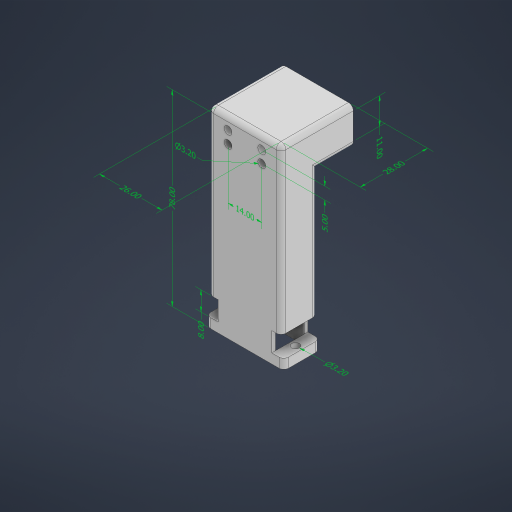
# Autodesk Inventor part: attachment of brush
Saved by Autodesk Inventor 2024.2 (Build 282272000, 272)
## iProperties
Created: 2024-03-09
Part Number: attachment of brush
Material: Generic
Document SubType Name: Modeling
Designer: seifs
Density: 1 g/cm^3
Appearance: Default
Author: seifs
Autodesk Inventor part; units mm, degrees
ref_plane "YZ Plane" through (0, 0, 0) normal (1, 0, 0) x (0, 1, 0)
ref_plane "XZ Plane" through (0, 0, 0) normal (0, 1, 0) x (-1, 0, 0)
ref_plane "XY Plane" through (0, 0, 0) normal (0, 0, 1) x (1, 0, 0)
sketch "Sketch1" plane through (0, 0, 0) normal (0, 0, 1) x (1, 0, 0)
  line L0 (-15, 7.5) -> (15, 7.5)
  line L1 (15, 7.5) -> (15, -7.5)
  line L2 (15, -7.5) -> (-15, -7.5)
  line L3 (-15, -7.5) -> (-15, 7.5)
  line L4 (-15, 7.5) -> (15, -7.5) construction
  line L5 (15, 7.5) -> (-15, -7.5) construction
  line L6 (-15, 0) -> (-7, 0) construction
  line L7 (-7, 0) -> (-7, -2.5) construction
  line L8 (0, 7.5) -> (0, -7.5) construction
  circle A0 centre (-7, -2.5) radius 1.6
  line L9 (0, -7.5) -> (0, 7.5) construction
  circle A1 centre (-7, 2.5) radius 1.6
  circle A2 centre (7, -2.5) radius 1.6
  circle A3 centre (7, 2.5) radius 1.6
  line L10 (7, 2.5) -> (-7, 2.5) construction
  point P0 (0, 0)
  dimension "d0" = 30
  dimension "d1" = 15
  dimension "d3" = 2.5
  dimension "d4" = 3.2
  dimension "d11" = 14
  constraints: 22 end point, 5 midpoint, 5 symmetric about line, 4 centre point, 3 horizontal, 2 parallel, 2 perpendicular, 1 coincident, 3 other
  measures "d0" distance of L1.end L2.end
  measures "d1" distance of L0.end L1.end
  measures "d3" distance of L6.end L7.end
  measures "d4" diameter of A0
  measures "d11" distance of L10.start L10.end
extrude "Extrusion1" add sketch "Sketch1" along normal blind 30
sketch "Sketch2" plane through (-15, -7.5, 0) normal (0, -1, 0) x (1, 0, 0)
  line L0 (0, 30) -> (30, 30) projected
  line L1 (0, 30) -> (30, 30)
  line L2 (30, 30) -> (30, 15)
  line L3 (30, 15) -> (0, 15)
  line L4 (0, 15) -> (0, 30)
  point P0 (15, 0)
  dimension "d7" = 30
  dimension "d8" = 15
  constraints: 8 end point, 2 parallel, 1 horizontal, 1 perpendicular
  measures "d7" distance of L2.end L3.end
  measures "d8" distance of L1.end L2.end
extrude "Extrusion2" add sketch "Sketch2" along normal blind 50
sketch "Sketch3" plane through (-15, -57.5, 0) normal (0, -1, 0) x (1, 0, 0)
  line L0 (0, 15) -> (30, 15) projected
  line L1 (15, 15) -> (15, 22.5) construction
  line L2 (15, 22.5) -> (3.85, 22.5) construction
  line L3 (15, 22.5) -> (26.15, 22.5) construction
  line L4 (3.85, 28.45) -> (26.15, 28.45)
  line L5 (26.15, 28.45) -> (26.15, 16.55)
  line L6 (26.15, 16.55) -> (3.85, 16.55)
  line L7 (3.85, 16.55) -> (3.85, 28.45)
  line L8 (3.85, 28.45) -> (26.15, 16.55) construction
  line L9 (26.15, 28.45) -> (3.85, 16.55) construction
  line L10 (0, 30) -> (30, 30)
  line L11 (30, 30) -> (30, 15)
  line L12 (30, 15) -> (0, 15)
  line L13 (0, 15) -> (0, 30)
  line L14 (0, 30) -> (30, 15) construction
  line L15 (30, 30) -> (0, 15) construction
  point P0 (15, 0)
  dimension "d12" = 7.5
  dimension "d14" = 11.15
  dimension "d15" = 11.15
  dimension "d19" = 22.3
  dimension "d20" = 11.9
  dimension "d21" = 15
  constraints: 30 end point, 5 midpoint, 4 horizontal, 4 parallel, 2 perpendicular, 1 vertical
  measures "d12" distance of L1.end L1.start
  measures "d14" distance of L1.end L2.end
  measures "d15" distance of L1.end L3.end
  measures "d19" distance of L5.end L6.end
  measures "d20" distance of L4.end L5.end
  measures "d21" distance of L10.end L0.end
extrude "Extrusion3" add sketch "Sketch3" along normal blind 15
sketch "Sketch4" plane through (-15, -72.5, 0) normal (0, -1, 0) x (1, 0, 0)
  line L0 (30, 30) -> (0, 30) projected
  line L1 (0, 30) -> (3.85, 30)
  line L2 (3.85, 30) -> (3.85, 15)
  line L3 (3.85, 15) -> (0, 15)
  line L4 (0, 15) -> (0, 30)
  line L5 (30, 0) -> (30, 30) projected
  line L6 (30, 30) -> (26.15, 30)
  line L7 (26.15, 30) -> (26.15, 15)
  line L8 (26.15, 15) -> (30, 15)
  line L9 (30, 15) -> (30, 30)
  point P0 (15, 0)
  dimension "d24" = 15
  dimension "d25" = 15
  constraints: 16 end point, 4 parallel, 2 horizontal, 2 perpendicular
  measures "d24" distance of L1.end L2.end
  measures "d25" distance of L7.end L6.end
extrude "Extrusion4" cut sketch "Sketch4" against normal blind 12
sketch "Sketch5" plane through (-11.15, -72.5, 15) normal (-1, 0, 0) x (0, 0, 1)
  line L0 (13.45, 0) -> (15, 0) projected
  line L1 (15, 0) -> (0, 0)
  line L2 (0, 0) -> (0, 4)
  line L3 (0, 4) -> (15, 4)
  line L4 (15, 4) -> (15, 0)
  point P0 (-15, 72.5)
  point P1 (13.45, 0)
  dimension "d28" = 15
  dimension "d29" = 4
  constraints: 8 end point, 2 parallel, 1 horizontal, 1 perpendicular
  measures "d28" distance of L2.end L3.end
  measures "d29" distance of L1.end L2.end
extrude "Extrusion5" add sketch "Sketch5" along normal blind 5
sketch "Sketch6" plane through (-15, -72.5, 0) normal (0, -1, 0) x (1, 0, 0)
  line L0 (3.85, 28.45) -> (3.85, 16.55) projected
  circle A0 centre (1.5, 22.5) radius 1.6
  line L1 (26.15, 28.45) -> (3.85, 28.45) construction
  line L2 (15, 28.45) -> (15, 16.55) construction
  line L3 (3.85, 16.55) -> (26.15, 16.55) construction
  point P0 (15, 0)
  dimension "d33" = 3.2
  dimension "d56" = 13.5
  constraints: 2 end point, 2 midpoint, 1 centre point
  measures "d33" diameter of A0
  measures "d56" distance from line of L2 A0.centre
extrude "Extrusion6" cut sketch "Sketch6" against normal blind 4
mirror "Mirror1" about plane through (0, 0, 0) normal (1, 0, 0) of "Extrusion5"
mirror "Mirror2" about plane through (0, 0, 0) normal (1, 0, 0) of "Extrusion6"
fillet "Fillet1" radius 2 13 edges at (15, -7.5, 7.5) (15, 7.5, 15) (-15, -7.5, 7.5) (-15, 7.5, 15) (-15, -34, 15) (15, -34, 15) (-15, -26.5, 30) (15, -26.5, 30) (0, 7.5, 30) (16.15, -70.5, 15) (-16.15, -70.5, 15) (-16.15, -70.5, 30) (16.15, -70.5, 30)
body "Solid1"
